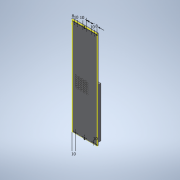
# Autodesk Inventor part: LeftBoxCover
Saved by Autodesk Inventor 2020 (Build 240168000, 168)
## iProperties
Created: 2019-06-03
Part Number: LeftBoxCover
Material: Generic
Document SubType Name: Modeling
Designer: LillaHunden
Density: 1 g/cm^3
Appearance: Default
Author: LillaHunden
Autodesk Inventor part; units mm, degrees
ref_plane "YZ Plane" through (0, 0, 0) normal (1, 0, 0) x (0, 1, 0)
ref_plane "XZ Plane" through (0, 0, 0) normal (0, 1, 0) x (-1, 0, 0)
ref_plane "XY Plane" through (0, 0, 0) normal (0, 0, 1) x (1, 0, 0)
sketch "Sketch1" plane through (0, 0, 0) normal (0, 0, 1) x (1, 0, 0)
  line L0 (67, 4) -> (76.9823, 4) construction
  line L1 (76.9823, 4) -> (76.9823, 12) construction
  line L2 (0, 12) -> (76.9823, 12) construction
  line L3 (0, 0) -> (0, 12) construction
  line L4 (67, 0) -> (0, 0) construction
  line L5 (67, 0) -> (67, 4) construction
  line L6 (67, -280) -> (67, -276) construction
  line L7 (67, -276) -> (0, -276) construction
  line L8 (0, -276) -> (0, -288) construction
  line L9 (76.9823, -288) -> (0, -288) construction
  line L10 (76.9823, -280) -> (76.9823, -288) construction
  line L11 (76.9823, -280) -> (67, -280) construction
  line L12 (76.9823, 12) -> (0, 12)
  line L13 (0, 12) -> (0, -288)
  line L14 (0, -288) -> (76.9823, -288)
  line L15 (76.9823, -288) -> (76.9823, 12)
  circle A0 centre (10, -284) radius 1.2295 projected
  circle A1 centre (66.9823, -284) radius 1.2295 projected
  circle A2 centre (38.4912, -284) radius 1.2295 projected
  constraints: 8 end point, 2 parallel, 1 horizontal, 1 perpendicular
extrude "Extrusion1" add sketch "Sketch1" along normal blind 12 contours L15 L14 L13 L12 | A0 | A1 | A2
sketch "Sketch2" plane through (0, 0, 0) normal (0, 0, -1) x (-1, 0, 0)
  line L0 (-76.9823, -280) -> (-67, -280) construction
  line L1 (-67, -276) -> (0, -276) construction
  line L2 (-67, -280) -> (-67, -276) construction
  line L3 (0, -275.9) -> (-67.1, -275.9)
  line L4 (-67.1, -275.9) -> (-67.1, -279.9)
  line L5 (-67.1, -279.9) -> (-76.9823, -279.9)
  line L6 (0, 12) -> (0, -288) projected
  line L7 (-76.9823, 12) -> (0, 12) projected
  line L8 (-76.9823, -288) -> (-76.9823, 12) projected
  line L9 (0, -288) -> (-76.9823, -288) projected
  point P0 (0, 0)
  dimension "d2" = 0.1
  constraints: 6 end point, 2 other
  measures "d2" distance between parallel lines of L1 L3
extrude "Extrusion2" cut sketch "Sketch2" against normal blind 8 contours L6 L9 L8 L5 L4 L3
sketch "Sketch3" plane through (0, 0, 0) normal (0, 0, -1) x (-1, 0, 0)
  line L0 (-67, 4) -> (-76.9823, 4) construction
  line L1 (-67, 0) -> (0, 0) construction
  line L2 (-67, 0) -> (-67, 4) construction
  line L3 (-76.9823, 3.9) -> (-67.1, 3.9)
  line L4 (-67.1, 3.9) -> (-67.1, -0.1)
  line L5 (-67.1, -0.1) -> (0, -0.1)
  line L6 (-67.1, -275.9) -> (0, -275.9) projected
  line L7 (0, 12) -> (0, -275.9) projected
  line L8 (-76.9823, 12) -> (0, 12) projected
  line L9 (-76.9823, -279.9) -> (-76.9823, 12) projected
  line L10 (-76.9823, -279.9) -> (-67.1, -279.9) projected
  line L11 (-67.1, -279.9) -> (-67.1, -275.9) projected
  point P0 (0, -0.1)
  dimension "d5" = 0.1
  constraints: 6 end point, 2 other
  measures "d5" distance between parallel lines of L0 L3
extrude "Extrusion3" cut sketch "Sketch3" against normal up to surface (8 mm away) contours L9 L8 L7 L5 L4 L3
sketch "Sketch4" plane through (76.9823, -288, 12) normal (1, 0, 0) x (0, 0, -1)
  line L0 (4, 291.9) -> (4, 300) projected
  line L1 (12, 8.1) -> (12, 291.9) projected
  line L2 (4, 291.9) -> (12, 291.9)
  line L3 (12, 291.9) -> (12, 161.7)
  line L4 (12, 161.7) -> (4, 161.7)
  line L5 (4, 161.7) -> (4, 291.9)
  line L6 (197, 162) -> (4, 162) construction
  point P0 (12, 288)
  dimension "d8" = 0.3
  constraints: 8 end point, 2 parallel, 1 horizontal, 1 perpendicular, 1 point on line
  measures "d8" distance between parallel lines of L6 L4
ref_plane "Work Plane1" through (48, -120, -184.25) normal (-1, 0, 0) x (0, 0, 1)
extrude "Extrusion4" cut sketch "Sketch4" against normal up to surface (28.9823 mm away) draft 0.3
sketch "Sketch5" plane through (48, -126.4518, 8.1518) normal (1, 0, 0) x (0, 0, -1)
  arc A0 (6.828, 119.8758) -> (6.828, 114.6758) centre (6.828, 117.2758) ccw construction
  line L0 (6.828, 119.8758) -> (21.628, 119.8758) construction
  line L1 (21.628, 114.6758) -> (6.828, 114.6758) construction
  arc A1 (6.828, 72.7358) -> (6.828, 67.5358) centre (6.828, 70.1358) ccw construction
  line L2 (21.628, 67.5358) -> (6.828, 67.5358) construction
  line L3 (6.828, 72.7358) -> (21.628, 72.7358) construction
  line L4 (21.628, 113.1758) -> (6.828, 113.1758)
  arc A2 (6.828, 121.3758) -> (6.828, 113.1758) centre (6.828, 117.2758) ccw
  line L5 (6.828, 121.3758) -> (21.628, 121.3758)
  line L6 (21.628, 66.0358) -> (6.828, 66.0358)
  arc A3 (6.828, 74.2358) -> (6.828, 66.0358) centre (6.828, 70.1358) ccw
  line L7 (6.828, 74.2358) -> (21.628, 74.2358)
  line L8 (8.1518, 126.3518) -> (8.1518, 0) projected
  line L9 (8.1518, 113.1758) -> (8.1518, 121.3758)
  line L10 (8.1518, 74.2358) -> (8.1518, 66.0358)
  point P0 (8.1518, 126.4518)
  point P1 (8.1518, 66.0358)
  point P2 (8.1518, 74.2358)
  dimension "d11" = 1.5
  dimension "d12" = 1.5
  constraints: 12 end point, 8 point on line, 4 point on circle, 2 centre point, 4 other
  measures "d11" radial gap between concentric circles of A0 A2
  measures "d12" radial gap between concentric circles of A1 A3
extrude "Extrusion5" cut sketch "Sketch5" against normal blind 6
sketch "Sketch6" plane through (48, -126.4518, 8.1518) normal (1, 0, 0) x (0, 0, -1)
  line L0 (193.1518, 6.4518) -> (0.1518, 6.4518) construction
  line L1 (0.1518, 6.4518) -> (0.1518, 0.4518) construction
  line L2 (193.1518, 0.4518) -> (0.1518, 0.4518) construction
  line L3 (193.1518, 6.4518) -> (193.1518, 0.4518) construction
  line L4 (0.1518, 10.4518) -> (193.1518, 10.4518) construction
  line L5 (0.1518, 0.4518) -> (193.1518, 0.4518) construction
  line L6 (0.1518, 0.1518) -> (0, 0) projected
  line L7 (8.1518, 66.0358) -> (8.1518, 0) projected
  line L8 (0, 0) -> (8.1518, 0)
  line L9 (8.1518, 0) -> (8.1518, 10.7518)
  line L10 (8.1518, 10.7518) -> (0, 10.7518)
  line L11 (0, 10.7518) -> (0, 0)
  point P0 (8.1518, 126.4518)
  dimension "d15" = 0.3
  constraints: 8 end point, 2 parallel, 1 horizontal, 1 perpendicular, 1 point on line
  measures "d15" distance between parallel lines of L10 L4
extrude "Extrusion6" cut sketch "Sketch6" against normal through all
sketch "Sketch7" plane through (0, -275.9, 0) normal (0, -1, 0) x (1, 0, 0)
  point P0 (56.9823, 2.6)
  point P1 (46.9823, 2.6)
  point P2 (30, 2.6)
  point P3 (20, 2.6)
hole "Hole1" at (56.9823, -275.9, 2.6) at (46.9823, -275.9, 2.6) at (30, -275.9, 2.6) at (20, -275.9, 2.6) direction (0, 1, 0) diameter 2.459 depth 8 tip angle 120 thread size "M3x0.5" class "6H" standard "ISO Metric profile"
sketch "Sketch9" plane through (0, 0, 12) normal (0, 0, 1) x (1, 0, 0)
  line L0 (0, 12) -> (0, -288) projected
  line L1 (76.9823, -288) -> (76.9823, 12) projected
  line L2 (76.9823, -280) -> (76.9823, -288) construction
  line L3 (50.2323, -288) -> (43.7323, -288) construction
  line L4 (33.25, -288) -> (26.75, -288) construction
  line L5 (43.7323, -288) -> (33.25, -288) construction
  line L6 (0, -288) -> (76.9823, -288) construction
  point P0 (0, 0)
  point P1 (66.9823, -284)
  point P2 (10, -284)
  point P3 (38.4912, -284)
  point P4 (76.9823, -284)
  point P5 (38.4912, -288)
  dimension "d37" = 10
  dimension "d38" = 10
  constraints: 3 horizontal alignment, 2 end point, 2 midpoint, 1 collinear, 1 vertical alignment
  measures "d37" distance from line of L0 point (10, -284)
  measures "d38" distance from line of L1 point (66.982, -284)
sketch "Sketch10" plane through (0, 0, 12) normal (0, 0, 1) x (1, 0, 0)
  point P0 (66.9823, -284)
  point P1 (10, -284)
  point P2 (38.4912, -284)
hole "Hole3" at (66.9823, -284, 12) at (10, -284, 12) at (38.4912, -284, 12) direction (0, 0, -1) diameter 3.4 depth 4
sketch "Sketch11" plane through (0, 0, 12) normal (0, 0, 1) x (1, 0, 0)
  line L0 (24.2323, -158) -> (25.6073, -155.6184)
  line L1 (25.6073, -155.6184) -> (28.3573, -155.6184)
  line L2 (28.3573, -155.6184) -> (29.7323, -158)
  line L3 (29.7323, -158) -> (28.3573, -160.3816)
  line L4 (28.3573, -160.3816) -> (25.6073, -160.3816)
  line L5 (25.6073, -160.3816) -> (24.2323, -158)
  line L6 (19.3148, -160.8816) -> (20.6898, -158.5)
  line L7 (20.6898, -158.5) -> (23.4398, -158.5)
  line L8 (23.4398, -158.5) -> (24.8148, -160.8816)
  line L9 (24.8148, -160.8816) -> (23.4398, -163.2631)
  line L10 (23.4398, -163.2631) -> (20.6898, -163.2631)
  line L11 (20.6898, -163.2631) -> (19.3148, -160.8816)
  line L12 (19.3148, -155.1184) -> (20.6898, -152.7369)
  line L13 (20.6898, -152.7369) -> (23.4398, -152.7369)
  line L14 (23.4398, -152.7369) -> (24.8148, -155.1184)
  line L15 (24.8148, -155.1184) -> (23.4398, -157.5)
  line L16 (23.4398, -157.5) -> (20.6898, -157.5)
  line L17 (20.6898, -157.5) -> (19.3148, -155.1184)
  line L18 (24.2323, -152.2369) -> (25.6073, -149.8553)
  line L19 (25.6073, -149.8553) -> (28.3573, -149.8553)
  line L20 (28.3573, -149.8553) -> (29.7323, -152.2369)
  line L21 (29.7323, -152.2369) -> (28.3573, -154.6184)
  line L22 (28.3573, -154.6184) -> (25.6073, -154.6184)
  line L23 (25.6073, -154.6184) -> (24.2323, -152.2369)
  line L24 (24.2323, -163.7631) -> (25.6073, -161.3816)
  line L25 (25.6073, -161.3816) -> (28.3573, -161.3816)
  line L26 (28.3573, -161.3816) -> (29.7323, -163.7631)
  line L27 (29.7323, -163.7631) -> (28.3573, -166.1447)
  line L28 (28.3573, -166.1447) -> (25.6073, -166.1447)
  line L29 (25.6073, -166.1447) -> (24.2323, -163.7631)
  line L30 (19.3148, -149.3553) -> (20.6898, -146.9737)
  line L31 (20.6898, -146.9737) -> (23.4398, -146.9737)
  line L32 (23.4398, -146.9737) -> (24.8148, -149.3553)
  line L33 (24.8148, -149.3553) -> (23.4398, -151.7369)
  line L34 (23.4398, -151.7369) -> (20.6898, -151.7369)
  line L35 (20.6898, -151.7369) -> (19.3148, -149.3553)
  line L36 (24.2323, -152.2369) -> (22.9163, -152.2369) construction
  line L37 (18.3573, -160.3816) -> (15.6073, -160.3816)
  line L38 (15.6073, -160.3816) -> (14.2323, -158)
  line L39 (14.2323, -158) -> (15.6073, -155.6184)
  line L40 (19.7323, -158) -> (18.3573, -160.3816)
  line L41 (15.6073, -155.6184) -> (18.3573, -155.6184)
  line L42 (18.3573, -155.6184) -> (19.7323, -158)
  line L43 (9.3148, -155.1184) -> (10.6898, -152.7369)
  line L44 (13.4398, -152.7369) -> (14.8148, -155.1184)
  line L45 (14.8148, -155.1184) -> (13.4398, -157.5)
  line L46 (13.4398, -157.5) -> (10.6898, -157.5)
  line L47 (10.6898, -157.5) -> (9.3148, -155.1184)
  line L48 (10.6898, -152.7369) -> (13.4398, -152.7369)
  line L49 (13.4398, -151.7369) -> (10.6898, -151.7369)
  line L50 (15.6073, -154.6184) -> (14.2323, -152.2369)
  line L51 (10.6898, -151.7369) -> (9.3148, -149.3553)
  line L52 (9.3148, -149.3553) -> (10.6898, -146.9737)
  line L53 (10.6898, -146.9737) -> (13.4398, -146.9737)
  line L54 (14.8148, -149.3553) -> (13.4398, -151.7369)
  line L55 (14.2323, -152.2369) -> (15.6073, -149.8553)
  line L56 (18.3573, -154.6184) -> (15.6073, -154.6184)
  line L57 (13.4398, -146.9737) -> (14.8148, -149.3553)
  line L58 (19.7323, -152.2369) -> (18.3573, -154.6184)
  line L59 (15.6073, -149.8553) -> (18.3573, -149.8553)
  line L60 (18.3573, -149.8553) -> (19.7323, -152.2369)
  line L61 (14.2323, -152.2369) -> (12.9163, -152.2369) construction
  line L62 (15.6073, -161.3816) -> (18.3573, -161.3816)
  line L63 (13.4398, -158.5) -> (14.8148, -160.8816)
  line L64 (18.3573, -161.3816) -> (19.7323, -163.7631)
  line L65 (19.7323, -163.7631) -> (18.3573, -166.1447)
  line L66 (18.3573, -166.1447) -> (15.6073, -166.1447)
  line L67 (14.2323, -163.7631) -> (15.6073, -161.3816)
  line L68 (15.6073, -166.1447) -> (14.2323, -163.7631)
  line L69 (10.6898, -158.5) -> (13.4398, -158.5)
  line L70 (9.3148, -160.8816) -> (10.6898, -158.5)
  line L71 (13.4398, -163.2631) -> (10.6898, -163.2631)
  line L72 (10.6898, -163.2631) -> (9.3148, -160.8816)
  line L73 (14.8148, -160.8816) -> (13.4398, -163.2631)
  line L74 (76.9823, -288) -> (76.9823, 12) projected
  line L75 (76.9823, -158) -> (13.1534, -158) construction
  line L76 (0, -288) -> (76.9823, -288) projected
  point P0 (0, 0)
  point P1 (26.9823, -158)
  point P2 (22.0648, -160.8816)
  point P3 (22.0648, -155.1184)
  point P4 (26.9823, -152.2369)
  point P5 (26.9823, -163.7631)
  point P6 (22.0648, -149.3553)
  point P7 (16.9823, -158)
  point P8 (12.0648, -155.1184)
  point P9 (12.0648, -149.3553)
  point P10 (16.9823, -152.2369)
  point P11 (16.9823, -163.7631)
  point P12 (12.0648, -160.8816)
  dimension "d46" = 5.5
  dimension "d51" = 5.5
  dimension "d52" = 5.5
  dimension "d53" = 5.5
  dimension "d54" = 5.5
  dimension "d55" = 5.5
  dimension "d56" = 1
  dimension "d57" = 1
  dimension "d58" = 1
  dimension "d59" = 1
  dimension "d65" = 10
  dimension "honeycombYdir" = 130
  dimension "HoneycombZDir" = 50
  constraints: 150 end point, 6 horizontal alignment, 4 vertical alignment, 3 horizontal, 2 point on line, 1 collinear, 158 other
  measures "d46" distance of L2.end L0.start
  measures "d51" distance of L8.end L6.start
  measures "d52" distance of L14.end L12.start
  measures "d53" distance of L20.end L18.start
  measures "d54" distance of L26.end L24.start
  measures "d55" distance of L32.end L30.start
  measures "d56" distance between parallel lines of L13 L34
  measures "d57" distance between parallel lines of L7 L16
  measures "d58" distance between parallel lines of L1 L22
  measures "d59" distance between parallel lines of L25 L4
  measures "d65" distance of point (26.982, -158) point (16.982, -158)
  measures "honeycombYdir" distance between parallel lines of L76 L75
  measures "HoneycombZDir" distance from line of L74 point (26.982, -158)
extrude "Extrusion8" cut sketch "Sketch11" against normal through all
pattern_linear "Rectangular Pattern1" count 2 spacing 20 along (1, 0, 0) count 2 spacing 17 along (0, 1, 0) of "Extrusion8"
sketch "Sketch13" plane through (0, 0, 12) normal (0, 0, 1) x (1, 0, 0)
  line L0 (76.9823, 3.9) -> (76.9823, 12) projected
  line L1 (0, 12) -> (0, -288) projected
  line L2 (33.4912, 7.95) -> (43.4912, 7.95) construction
  line L3 (76.9823, 12) -> (0, 12) projected
  point P0 (0, 0)
  point P1 (68.9823, 7.95)
  point P2 (58.9823, 7.95)
  point P3 (18, 7.95)
  point P4 (8, 7.95)
  point P5 (76.9823, 7.95)
  point P6 (38.4912, 7.95)
  point P7 (38.4912, 12)
  dimension "d84" = 10
  dimension "d85" = 8
  dimension "d87" = 10
  dimension "d88" = 10
  dimension "d89" = 8
  constraints: 6 horizontal alignment, 3 midpoint, 2 end point, 1 horizontal, 1 vertical alignment
  measures "d84" distance of point (58.982, 7.95) point (68.982, 7.95)
  measures "d85" distance of point (76.982, 7.95) point (68.982, 7.95)
  measures "d87" distance of L2.start L2.end
  measures "d88" distance of point (8, 7.95) point (18, 7.95)
  measures "d89" distance from line of L1 point (8, 7.95)
equation "\"d57\" = d56"
equation "\"d58\" = d56"
equation "\"d59\" = d56"
body "Solid1"
